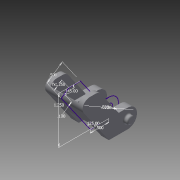
# Autodesk Inventor part: LegV3
Saved by Autodesk Inventor 2014 (Build 180170000, 170)
## iProperties
Created: 2014-04-25
Part Number: LegV3
Material: Generic
Document SubType Name: Modeling
Designer: Max
Density: 1 g/cm^3
Appearance: Default
Author: Max
Autodesk Inventor part; units mm, degrees
ref_plane "YZ Plane" through (0, 0, 0) normal (1, 0, 0) x (0, 1, 0)
ref_plane "XZ Plane" through (0, 0, 0) normal (0, 1, 0) x (-1, 0, 0)
ref_plane "XY Plane" through (0, 0, 0) normal (0, 0, 1) x (1, 0, 0)
sketch "Sketch1" plane through (0, 0, 0) normal (1, 0, 0) x (0, 1, 0)
  circle A0 centre (0, 0) radius 2.54
  circle A1 centre (0, 0) radius 6.35
  line L0 (-6.35, 0) -> (-6.35, 12.7)
  line L1 (-6.35, 12.7) -> (21.7578, 32.3813)
  line L2 (21.7578, 32.3813) -> (25.4, 27.1797)
  line L3 (25.4, 27.1797) -> (25.4, 19.4278)
  line L4 (25.4, 19.4278) -> (6.35, 6.0888)
  line L5 (6.35, 0) -> (6.35, 6.0888)
  line L6 (23.2147, 30.3006) -> (-6.35, 9.5992)
  line L7 (6.35, 0) -> (6.35, 18.4919)
  line L8 (6.35, 18.4919) -> (4.8931, 20.5725)
  dimension "d0" = 5.08
  dimension "d1" = 12.7
  dimension "d2" = 12.7
  dimension "d3" = 145
  dimension "d5" = 125
  dimension "d6" = 31.75
  dimension "d7" = 12.7
  dimension "d8" = 6.35
  dimension "d15" = 2.54
  constraints: 18 end point, 4 point on line, 3 perpendicular, 3 tangent, 2 centre point, 2 coincident, 2 parallel, 2 point on circle, 1 collinear, 1 vertical
  measures "d0" diameter of A0
  measures "d1" diameter of A1
  measures "d2" distance of L0.start L0.end
  measures "d3" angle of L3 L2
  measures "d5" angle of L0 L1
  measures "d6" horizontal distance of L0.start L3.end
  measures "d7" distance between parallel lines of L1 L4
  measures "d8" distance from line of L1 L2.end
  measures "d15" distance between parallel lines of L1 L6
extrude "Extrusion1" add sketch "Sketch1" along normal mid plane 25.4
extrude "Extrusion2" add sketch "Sketch1" along normal mid plane 30.48 contours A0
fillet "Fillet1" radius 4.7625 3 edges at (0, 25.4, 27.1797) (0, 21.7578, 32.3813) (0, 25.4, 19.4278)
fillet "Fillet2" radius 0.7937 4 edges at (15.24, -2.54, 0) (12.7, -2.54, 0) (-15.24, -2.54, 0) (-12.7, -2.54, 0)
extrude "Extrusion3" cut sketch "Sketch1" along normal mid plane 19.05 contours L7 L6 L2 L3 L4
extrude "Extrusion4" cut sketch "Sketch1" along normal mid plane 15.24 contours A0 | A1 | A1 L0 L6 L7 L5 | L0 L1 L8 L6
equation "\"d8\" = 0.5 * d7"
body "Solid1"
